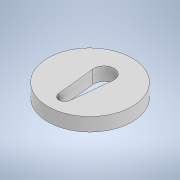
# Autodesk Inventor part: Ventil Scheibe
Saved by Autodesk Inventor 2022.2 (Build 262287000, 287)
## iProperties
Created: 2022-04-20
Part Number: Ventil Scheibe
Material: Generic
Document SubType Name: Modeling
Designer: Michel Esteves
Density: 1 g/cm^3
Appearance: Default
Author: Michel Esteves
## iProperties of the stored document Ventil Scheibe_3DPrint.ipt
Created: 2022-04-20
Part Number: Ventil Scheibe_3DPrint
Material: Generic
Document SubType Name: Modeling
Designer: Michel Esteves
Density: 1 g/cm^3
Appearance: Default
Author: Michel Esteves
Autodesk Inventor part; units mm, degrees
ref_plane "YZ Plane" through (0, 0, 0) normal (1, 0, 0) x (0, 1, 0)
ref_plane "XZ Plane" through (0, 0, 0) normal (0, 1, 0) x (-1, 0, 0)
ref_plane "XY Plane" through (0, 0, 0) normal (0, 0, 1) x (1, 0, 0)
sketch "Sketch1" plane through (0, 0, 0) normal (0, 1, 0) x (-1, 0, 0)
  circle A0 centre (0, 0) radius 20 construction
  circle A1 centre (0, 5) radius 15
  circle A2 centre (0, 0) radius 3.5
  circle A3 centre (0, 14) radius 2
  line L0 (-1.9885, 14.2143) -> (-3.4799, 0.375)
  line L1 (1.9885, 14.2143) -> (3.4799, 0.375)
  dimension "d0" = 40
  dimension "d1" = 30
  dimension "d2" = 7
  dimension "d3" = 4
  dimension "d4" = 19.5
  constraints: 5 tangent, 4 centre point, 4 end point, 4 point on circle, 2 coincident, 2 vertical alignment
  measures "d0" diameter of A0
  measures "d1" diameter of A1
  measures "d2" diameter of A2
  measures "d3" diameter of A3
extrude "Extrusion1" add sketch "Sketch1" along normal blind 4.8
sketch "Sketch2" plane through (0, 4.8, 5) normal (0, 1, 0) x (1, 0, 0)
  arc A0 (-1.9885, -9.2143) -> (1.9885, -9.2143) centre (0, -9) ccw projected
  line L0 (1.9885, -9.2143) -> (3.4799, 4.625) projected
  arc A1 (3.4799, 4.625) -> (-3.4799, 4.625) centre (0, 5) ccw projected
  line L1 (-3.4799, 4.625) -> (-1.9885, -9.2143) projected
  circle A2 centre (0, 0) radius 15 projected
  arc A3 (-2.0879, -9.225) -> (2.0879, -9.225) centre (0, -9) ccw
  line L2 (2.0879, -9.225) -> (3.5793, 4.6143)
  arc A4 (3.5793, 4.6143) -> (-3.5793, 4.6143) centre (0, 5) ccw
  line L3 (-3.5793, 4.6143) -> (-2.0879, -9.225)
  dimension "d7" = 0.1
  constraints: 4 end point, 4 point on circle, 2 centre point, 3 other
  measures "d7" distance between parallel lines of L1 L3
extrude "Extrusion2" cut sketch "Sketch2" against normal through all contours L3 A4 L2 A3
body "Solid1"
